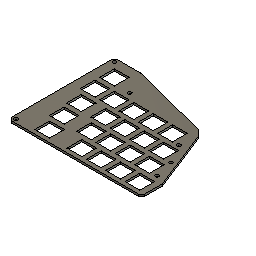
Main Plate v4 (Autodesk Fusion 360 design; units mm, degrees)
Autodesk Fusion 360 part; units mm, degrees
other "Base Mesh Feature1"
sketch "Sketch1" plane through (0, 0, 0) normal (0, 1, 0) x (1, 0, 0)
  line L0 (2.5, 38.25) -> (0, 40.75)
  line L1 (0, 40.75) -> (0, 136)
  line L2 (0, 136) -> (0, 138.5)
  line L3 (0, 138.5) -> (2.5, 138.5)
  line L4 (2.5, 138.5) -> (0, 136)
  line L5 (2.5, 138.5) -> (25, 138.5)
  line L6 (96.5, 117.5) -> (98.5, 117.5)
  line L7 (98.5, 117.5) -> (98.5, 119.5)
  line L8 (98.5, 119.5) -> (25, 138.5)
  line L9 (102, 112) -> (104, 112)
  line L10 (104, 112) -> (104, 114)
  line L11 (104, 114) -> (98.5, 119.5)
  line L12 (2.5, 38.25) -> (121.5, 38.25)
  line L13 (121.5, 38.25) -> (123.5, 38.25)
  line L14 (123.5, 38.25) -> (126, 38.25)
  line L15 (126, 38.25) -> (126, 40.75)
  line L16 (126, 40.75) -> (123.5, 38.25)
  line L17 (124, 58) -> (126, 58)
  line L18 (126, 58) -> (126, 40.75)
  line L19 (126, 58) -> (104, 114)
  dimension "d1" = 95.25
  dimension "d2" = 2.5
  dimension "d3" = 2.5
  dimension "d4" = 2
  dimension "d5" = 2
  dimension "d6" = 2
  dimension "d7" = 2
  dimension "d8" = 2.5
  dimension "d9" = 2.5
  constraint vertical L1
  constraint parallel L1 L2
  constraint perpendicular L2 L3
  constraint perpendicular L1 L5
  constraint perpendicular L1 L6
  constraint perpendicular L6 L7
  constraint perpendicular L7 L9
  constraint perpendicular L9 L10
  constraint horizontal L12
  constraint parallel L12 L13
  constraint parallel L13 L14
  constraint perpendicular L14 L15
  constraint parallel L13 L17
  constraint perpendicular L17 L18
  measures "d1" distance of L0.end L1.end
  measures "d2" distance of L1.end L2.end
  measures "d3" distance of L2.end L3.end
  measures "d4" distance of L6.start L6.end
  measures "d5" distance of L6.end L7.end
  measures "d6" distance of L9.start L9.end
  measures "d7" distance of L12.end L13.end
  measures "d8" distance of L13.end L14.end
  measures "d9" distance of L14.end L15.end
extrude "Extrude1" add sketch "Sketch1" against normal blind 2 contours L0 L1 L4 L5 L8 L11 L12 L13 L16 L18 L19
sketch "Sketch2" plane through (0, 0, 0) normal (0, 1, 0) x (-1, 0, 0)
  line L0 (-126, -40.75) -> (-126, -58)
  line L1 (-126, -58) -> (-104, -114)
  line L2 (-104, -114) -> (-98.5, -119.5)
  line L3 (-98.5, -119.5) -> (-25, -138.5)
  line L4 (-25, -138.5) -> (-2.5, -138.5)
  line L5 (-2.5, -138.5) -> (0, -136)
  line L6 (0, -136) -> (0, -40.75)
  line L7 (0, -40.75) -> (-2.5, -38.25)
  line L8 (-2.5, -38.25) -> (-123.5, -38.25)
  line L9 (-123.5, -38.25) -> (-126, -40.75)
  line L10 (-3.5, -40.125) -> (-3.5, -41.75)
  circle A0 centre (-3.5, -41.75) radius 1.625
  line L11 (0, -138.5) -> (-3.45, -138.5)
  line L12 (-3.45, -138.5) -> (-3.45, -135.05)
  circle A1 centre (-3.45, -135.05) radius 1.625
  dimension "d12" = 1.625
  dimension "d13" = 3.45
  dimension "d14" = 3.45
  dimension "d15" = 3.25
  constraint vertical L10
  constraint coincident L10.end A0.centre
  constraint coincident L10.start A0
  constraint parallel L4 L11
  constraint perpendicular L11 L12
  constraint coincident L12.end A1.centre
  measures "d12" distance of L10.start L10.end
  measures "d13" distance of L11.start L11.end
  measures "d14" distance of L11.end L12.end
  measures "d15" diameter of A1
extrude "Extrude2" cut sketch "Sketch2" against normal blind 2 contours A0 | A1
move_body "Move1" bodies 1 to x (1, 0, 0) y (0, 1, 0) z (0, 0, 1) at (0, 0, 38.25)
sketch "Sketch3" plane through (0, 0, 0) normal (0, 1, 0) x (-1, 0, 0)
  circle A0 centre (-3.45, -96.8) radius 1.625
  circle A1 centre (-3.5, -3.5) radius 1.625
  line L0 (-126, -2.5) -> (-126, -19.75)
  line L1 (-126, -19.75) -> (-104, -75.75)
  line L2 (-104, -75.75) -> (-98.5, -81.25)
  line L3 (-98.5, -81.25) -> (-25, -100.25)
  line L4 (-25, -100.25) -> (-2.5, -100.25)
  line L5 (-2.5, -100.25) -> (0, -97.75)
  line L6 (0, -97.75) -> (0, -2.5)
  line L7 (0, -2.5) -> (-2.5, 0)
  line L8 (-2.5, 0) -> (-123.5, 0)
  line L9 (-123.5, 0) -> (-126, -2.5)
  line L10 (-21.075, -3.85) -> (-35.075, -3.85)
  line L11 (-35.075, -3.85) -> (-35.075, -17.85)
  line L12 (-35.075, -17.85) -> (-21.075, -17.85)
  line L13 (-21.075, -17.85) -> (-21.075, -3.85)
  line L14 (-51, -3.85) -> (-51.5, -3.85)
  line L15 (-51.5, -3.85) -> (-65.5, -3.85)
  line L16 (-65.5, -3.85) -> (-65.5, -17.85)
  line L17 (-65.5, -17.85) -> (-51.5, -17.85)
  line L18 (-51.5, -17.85) -> (-51.5, -3.85)
  line L19 (-65.5, -3.85) -> (-83.85, -3.85)
  line L20 (-83.85, -3.85) -> (-69.85, -3.85)
  line L21 (-69.85, -3.85) -> (-69.85, -17.85)
  line L22 (-69.85, -17.85) -> (-83.85, -17.85)
  line L23 (-83.85, -17.85) -> (-83.85, -3.85)
  line L24 (-83.85, -3.85) -> (-102.2, -3.85)
  line L25 (-102.2, -3.85) -> (-88.2, -3.85)
  line L26 (-88.2, -3.85) -> (-88.2, -17.85)
  line L27 (-88.2, -17.85) -> (-102.2, -17.85)
  line L28 (-102.2, -17.85) -> (-102.2, -3.85)
  line L29 (-102.2, -3.85) -> (-120.55, -3.85)
  line L30 (-120.55, -3.85) -> (-106.55, -3.85)
  line L31 (-106.55, -3.85) -> (-106.55, -17.85)
  line L32 (-106.55, -17.85) -> (-120.55, -17.85)
  line L33 (-120.55, -17.85) -> (-120.55, -3.85)
  dimension "d18" = 14
  dimension "d19" = 14
  dimension "d20" = 0.5
  dimension "d21" = 14
  dimension "d22" = 14
  dimension "d23" = 18.35
  dimension "d24" = 14
  dimension "d25" = 14
  dimension "d26" = 18.35
  dimension "d27" = 14
  dimension "d28" = 14
  dimension "d29" = 18.35
  dimension "d30" = 14
  dimension "d31" = 14
  constraint horizontal L10
  constraint vertical L11
  constraint horizontal L12
  constraint vertical L13
  constraint horizontal L14
  constraint horizontal L15
  constraint vertical L16
  constraint horizontal L17
  constraint vertical L18
  constraint perpendicular L16 L19
  constraint horizontal L20
  constraint vertical L21
  constraint horizontal L22
  constraint vertical L23
  constraint perpendicular L23 L24
  constraint horizontal L25
  constraint vertical L26
  constraint horizontal L27
  constraint vertical L28
  constraint perpendicular L28 L29
  constraint horizontal L30
  constraint vertical L31
  constraint horizontal L32
  constraint vertical L33
  measures "d18" distance of L10.start L10.end
  measures "d19" distance of L10.start L12.end
  measures "d20" distance of L14.start L14.end
  measures "d21" distance of L14.end L15.end
  measures "d22" distance of L14.end L17.end
  measures "d23" distance of L15.end L19.end
  measures "d24" distance of L19.end L20.end
  measures "d25" distance of L19.end L22.end
  measures "d26" distance of L19.end L24.end
  measures "d27" distance of L24.end L25.end
  measures "d28" distance of L24.end L27.end
  measures "d29" distance of L24.end L29.end
  measures "d30" distance of L29.end L30.end
  measures "d31" distance of L29.end L32.end
extrude "Extrude3" cut sketch "Sketch3" against normal blind 2 contours L10 L11 L12 L13 | L15 L16 L17 L18 | L19 L20 L21 L22 L23 | L24 L25 L26 L27 L28 | L29 L30 L31 L32 L33
sketch "Sketch4" plane through (0, 0, 0) normal (0, 1, 0) x (1, 0, 0)
  line L0 (16.5, 21.725) -> (16.5, 22.225)
  line L1 (16.5, 22.225) -> (30.5, 22.225)
  line L2 (30.5, 22.225) -> (30.5, 36.225)
  line L3 (30.5, 36.225) -> (16.5, 36.225)
  line L4 (16.5, 36.225) -> (16.5, 22.225)
  line L5 (41.675, 21.725) -> (42.175, 21.725)
  line L6 (42.175, 21.725) -> (42.175, 22.225)
  line L7 (42.175, 22.225) -> (41.675, 22.225)
  line L8 (41.675, 22.225) -> (41.675, 21.725)
  line L9 (42.175, 22.225) -> (56.175, 22.225)
  line L10 (56.175, 22.225) -> (56.175, 36.225)
  line L11 (56.175, 36.225) -> (42.175, 36.225)
  line L12 (42.175, 36.225) -> (42.175, 22.225)
  line L13 (56.175, 22.225) -> (74.525, 22.225)
  line L14 (74.525, 22.225) -> (60.525, 22.225)
  line L15 (60.525, 22.225) -> (60.525, 36.225)
  line L16 (60.525, 36.225) -> (74.525, 36.225)
  line L17 (74.525, 36.225) -> (74.525, 22.225)
  line L18 (74.525, 22.225) -> (92.875, 22.225)
  line L19 (92.875, 22.225) -> (78.875, 22.225)
  line L20 (78.875, 22.225) -> (78.875, 36.225)
  line L21 (78.875, 36.225) -> (92.875, 36.225)
  line L22 (92.875, 36.225) -> (92.875, 22.225)
  line L23 (92.875, 22.225) -> (111.225, 22.225)
  line L24 (111.225, 22.225) -> (97.225, 22.225)
  line L25 (97.225, 22.225) -> (97.225, 36.225)
  line L26 (97.225, 36.225) -> (111.225, 36.225)
  line L27 (111.225, 36.225) -> (111.225, 22.225)
  line L28 (113.375, 23.75) -> (115.5, 23.75)
  circle A0 centre (115.5, 23.75) radius 1.625
  dimension "d34" = 0.5
  dimension "d35" = 14
  dimension "d36" = 14
  dimension "d37" = 0.5
  dimension "d38" = 0.5
  dimension "d39" = 14
  dimension "d40" = 14
  dimension "d41" = 18.35
  dimension "d42" = 14
  dimension "d43" = 14
  dimension "d44" = 18.35
  dimension "d45" = 14
  dimension "d46" = 14
  dimension "d47" = 18.35
  dimension "d48" = 14
  dimension "d49" = 14
  dimension "d50" = 2.125
  dimension "d51" = 3.25
  constraint vertical L0
  constraint horizontal L1
  constraint vertical L2
  constraint horizontal L3
  constraint vertical L4
  constraint horizontal L5
  constraint vertical L6
  constraint horizontal L7
  constraint vertical L8
  constraint horizontal L9
  constraint vertical L10
  constraint horizontal L11
  constraint vertical L12
  constraint perpendicular L10 L13
  constraint horizontal L14
  constraint vertical L15
  constraint horizontal L16
  constraint vertical L17
  constraint perpendicular L17 L18
  constraint horizontal L19
  constraint vertical L20
  constraint horizontal L21
  constraint vertical L22
  constraint perpendicular L22 L23
  constraint horizontal L24
  constraint vertical L25
  constraint horizontal L26
  constraint vertical L27
  constraint horizontal L28
  constraint coincident L28.end A0.centre
  measures "d34" distance of L0.start L0.end
  measures "d35" distance of L0.end L1.end
  measures "d36" distance of L0.end L3.end
  measures "d37" distance of L5.start L5.end
  measures "d38" distance of L5.start L7.end
  measures "d39" distance of L6.end L9.end
  measures "d40" distance of L6.end L11.end
  measures "d41" distance of L9.end L13.end
  measures "d42" distance of L13.end L14.end
  measures "d43" distance of L13.end L16.end
  measures "d44" distance of L13.end L18.end
  measures "d45" distance of L18.end L19.end
  measures "d46" distance of L18.end L21.end
  measures "d47" distance of L18.end L23.end
  measures "d48" distance of L23.end L24.end
  measures "d49" distance of L23.end L26.end
  measures "d50" distance of L28.start L28.end
  measures "d51" diameter of A0
extrude "Extrude4" cut sketch "Sketch4" against normal blind 2 contours L1 L2 L3 L4 | L9 L10 L11 L12 | L13 L14 L15 L16 L17 | L18 L19 L20 L21 L22 | L23 L24 L25 L26 L27 | A0
sketch "Sketch5" plane through (0, 0, 0) normal (0, 1, 0) x (-1, 0, 0)
  line L0 (-78.875, -22.225) -> (-78.875, -36.225)
  line L1 (-78.875, -36.225) -> (-92.875, -36.225)
  line L2 (-92.875, -36.225) -> (-92.875, -22.225)
  line L3 (-92.875, -22.225) -> (-78.875, -22.225)
  line L4 (-30.5, -22.225) -> (-16.5, -22.225)
  line L5 (-16.5, -22.225) -> (-16.5, -36.225)
  line L6 (-16.5, -36.225) -> (-30.5, -36.225)
  line L7 (-30.5, -36.225) -> (-30.5, -22.225)
  line L8 (-97.225, -22.225) -> (-97.225, -36.225)
  line L9 (-97.225, -36.225) -> (-111.225, -36.225)
  line L10 (-111.225, -36.225) -> (-111.225, -22.225)
  line L11 (-111.225, -22.225) -> (-97.225, -22.225)
  line L12 (-60.525, -22.225) -> (-60.525, -36.225)
  line L13 (-60.525, -36.225) -> (-74.525, -36.225)
  line L14 (-74.525, -36.225) -> (-74.525, -22.225)
  line L15 (-74.525, -22.225) -> (-60.525, -22.225)
  line L16 (-56.175, -22.225) -> (-42.175, -22.225)
  line L17 (-42.175, -22.225) -> (-42.175, -36.225)
  line L18 (-42.175, -36.225) -> (-56.175, -36.225)
  line L19 (-56.175, -36.225) -> (-56.175, -22.225)
  circle A0 centre (-115.5, -23.75) radius 1.625
  line L20 (-69.85, -3.85) -> (-69.85, -17.85)
  line L21 (-69.85, -17.85) -> (-83.85, -17.85)
  line L22 (-83.85, -17.85) -> (-83.85, -3.85)
  line L23 (-83.85, -3.85) -> (-69.85, -3.85)
  line L24 (-88.2, -3.85) -> (-88.2, -17.85)
  line L25 (-88.2, -17.85) -> (-102.2, -17.85)
  line L26 (-102.2, -17.85) -> (-102.2, -3.85)
  line L27 (-102.2, -3.85) -> (-88.2, -3.85)
  line L28 (-65.5, -3.85) -> (-51.5, -3.85)
  line L29 (-51.5, -3.85) -> (-51.5, -17.85)
  line L30 (-51.5, -17.85) -> (-65.5, -17.85)
  line L31 (-65.5, -17.85) -> (-65.5, -3.85)
  line L32 (-106.55, -3.85) -> (-106.55, -17.85)
  line L33 (-106.55, -17.85) -> (-120.55, -17.85)
  line L34 (-120.55, -17.85) -> (-120.55, -3.85)
  line L35 (-120.55, -3.85) -> (-106.55, -3.85)
  line L36 (-35.075, -3.85) -> (-21.075, -3.85)
  line L37 (-21.075, -3.85) -> (-21.075, -17.85)
  line L38 (-21.075, -17.85) -> (-35.075, -17.85)
  line L39 (-35.075, -17.85) -> (-35.075, -3.85)
  circle A1 centre (-3.45, -96.8) radius 1.625
  circle A2 centre (-3.5, -3.5) radius 1.625
  line L40 (-126, -2.5) -> (-126, -19.75)
  line L41 (-126, -19.75) -> (-104, -75.75)
  line L42 (-104, -75.75) -> (-98.5, -81.25)
  line L43 (-98.5, -81.25) -> (-25, -100.25)
  line L44 (-25, -100.25) -> (-2.5, -100.25)
  line L45 (-2.5, -100.25) -> (0, -97.75)
  line L46 (0, -97.75) -> (0, -2.5)
  line L47 (0, -2.5) -> (-2.5, 0)
  line L48 (-2.5, 0) -> (-123.5, 0)
  line L49 (-123.5, 0) -> (-126, -2.5)
  line L50 (-14.325, -39.6) -> (-14.325, -40.6)
  line L51 (-14.325, -40.6) -> (-28.325, -40.6)
  line L52 (-28.325, -40.6) -> (-28.325, -54.6)
  line L53 (-28.325, -54.6) -> (-14.325, -54.6)
  line L54 (-14.325, -54.6) -> (-14.325, -40.6)
  line L55 (-36.75, -39.6) -> (-37.25, -39.6)
  line L56 (-37.25, -39.6) -> (-37.25, -40.6)
  line L57 (-37.25, -40.6) -> (-36.75, -40.6)
  line L58 (-36.75, -40.6) -> (-36.75, -39.6)
  line L59 (-37.25, -40.6) -> (-51.25, -40.6)
  line L60 (-51.25, -40.6) -> (-51.25, -54.6)
  line L61 (-51.25, -54.6) -> (-37.25, -54.6)
  line L62 (-37.25, -54.6) -> (-37.25, -40.6)
  line L63 (-51.25, -40.6) -> (-69.6, -40.6)
  line L64 (-69.6, -40.6) -> (-55.6, -40.6)
  line L65 (-55.6, -40.6) -> (-55.6, -54.6)
  line L66 (-55.6, -54.6) -> (-69.6, -54.6)
  line L67 (-69.6, -54.6) -> (-69.6, -40.6)
  line L68 (-69.6, -40.6) -> (-87.95, -40.6)
  line L69 (-87.95, -40.6) -> (-73.95, -40.6)
  line L70 (-73.95, -40.6) -> (-73.95, -54.6)
  line L71 (-73.95, -54.6) -> (-87.95, -54.6)
  line L72 (-87.95, -54.6) -> (-87.95, -40.6)
  line L73 (-87.95, -40.6) -> (-106.3, -40.6)
  line L74 (-106.3, -40.6) -> (-92.3, -40.6)
  line L75 (-92.3, -40.6) -> (-92.3, -54.6)
  line L76 (-92.3, -54.6) -> (-106.3, -54.6)
  line L77 (-106.3, -54.6) -> (-106.3, -40.6)
  line L78 (-108.875, -41.25) -> (-111, -41.25)
  line L79 (-111, -41.25) -> (-112.5, -41.25)
  circle A3 centre (-112.5, -41.25) radius 1.625
  line L80 (-115.5, -23.75) -> (-117, -23.75)
  circle A4 centre (-117, -23.75) radius 1.625
  dimension "d54" = 1
  dimension "d55" = 14
  dimension "d56" = 14
  dimension "d57" = 0.5
  dimension "d58" = 1
  dimension "d59" = 14
  dimension "d60" = 14
  dimension "d61" = 18.35
  dimension "d62" = 14
  dimension "d63" = 14
  dimension "d64" = 18.35
  dimension "d65" = 14
  dimension "d66" = 14
  dimension "d67" = 18.35
  dimension "d68" = 14
  dimension "d69" = 14
  dimension "d70" = 2.125
  dimension "d71" = 1.5
  dimension "d72" = 3.25
  dimension "d73" = 1.5
  dimension "d74" = 3.25
  constraint vertical L50
  constraint horizontal L51
  constraint vertical L52
  constraint horizontal L53
  constraint vertical L54
  constraint horizontal L55
  constraint vertical L56
  constraint horizontal L57
  constraint vertical L58
  constraint horizontal L59
  constraint vertical L60
  constraint horizontal L61
  constraint vertical L62
  constraint perpendicular L60 L63
  constraint horizontal L64
  constraint vertical L65
  constraint horizontal L66
  constraint vertical L67
  constraint perpendicular L67 L68
  constraint horizontal L69
  constraint vertical L70
  constraint horizontal L71
  constraint vertical L72
  constraint perpendicular L72 L73
  constraint horizontal L74
  constraint vertical L75
  constraint horizontal L76
  constraint vertical L77
  constraint horizontal L78
  constraint parallel L78 L79
  constraint coincident L79.end A3.centre
  constraint coincident A0.centre L80.start
  constraint horizontal L80
  constraint coincident L80.end A4.centre
  measures "d54" distance of L50.start L50.end
  measures "d55" distance of L50.end L51.end
  measures "d56" distance of L50.end L53.end
  measures "d57" distance of L55.start L55.end
  measures "d58" distance of L55.start L57.end
  measures "d59" distance of L56.end L59.end
  measures "d60" distance of L56.end L61.end
  measures "d61" distance of L59.end L63.end
  measures "d62" distance of L63.end L64.end
  measures "d63" distance of L63.end L66.end
  measures "d64" distance of L63.end L68.end
  measures "d65" distance of L68.end L69.end
  measures "d66" distance of L68.end L71.end
  measures "d67" distance of L68.end L73.end
  measures "d68" distance of L73.end L74.end
  measures "d69" distance of L73.end L76.end
  measures "d70" distance of L78.start L78.end
  measures "d71" distance of L78.end L79.end
  measures "d72" diameter of A3
  measures "d73" distance of A0.centre L80.end
  measures "d74" diameter of A4
extrude "Extrude5" cut sketch "Sketch5" against normal blind 2 contours A0 A4 | A0 A4 | L51 L52 L53 L54 | L59 L60 L61 L62 | L63 L64 L65 L66 L67 | L68 L69 L70 L71 L72 | L73 L74 L75 L76 L77 | A3 picked at (-116.5388, -23.75) picked at (-118.049, -23.3238)
sketch "Sketch6" plane through (0, 0, 0) normal (0, 1, 0) x (-1, 0, 0)
  line L0 (-126, -2.5) -> (-126, -19.75)
  line L1 (-126, -19.75) -> (-104, -75.75)
  line L2 (-104, -75.75) -> (-98.5, -81.25)
  line L3 (-98.5, -81.25) -> (-25, -100.25)
  line L4 (-25, -100.25) -> (-2.5, -100.25)
  line L5 (-2.5, -100.25) -> (0, -97.75)
  line L6 (0, -97.75) -> (0, -2.5)
  line L7 (0, -2.5) -> (-2.5, 0)
  line L8 (-2.5, 0) -> (-123.5, 0)
  line L9 (-123.5, 0) -> (-126, -2.5)
  circle A0 centre (-3.5, -3.5) radius 1.625
  circle A1 centre (-3.45, -96.8) radius 1.625
  line L10 (-35.075, -3.85) -> (-21.075, -3.85)
  line L11 (-21.075, -3.85) -> (-21.075, -17.85)
  line L12 (-21.075, -17.85) -> (-35.075, -17.85)
  line L13 (-35.075, -17.85) -> (-35.075, -3.85)
  line L14 (-106.55, -3.85) -> (-106.55, -17.85)
  line L15 (-106.55, -17.85) -> (-120.55, -17.85)
  line L16 (-120.55, -17.85) -> (-120.55, -3.85)
  line L17 (-120.55, -3.85) -> (-106.55, -3.85)
  line L18 (-65.5, -3.85) -> (-51.5, -3.85)
  line L19 (-51.5, -3.85) -> (-51.5, -17.85)
  line L20 (-51.5, -17.85) -> (-65.5, -17.85)
  line L21 (-65.5, -17.85) -> (-65.5, -3.85)
  line L22 (-88.2, -3.85) -> (-88.2, -17.85)
  line L23 (-88.2, -17.85) -> (-102.2, -17.85)
  line L24 (-102.2, -17.85) -> (-102.2, -3.85)
  line L25 (-102.2, -3.85) -> (-88.2, -3.85)
  line L26 (-69.85, -3.85) -> (-69.85, -17.85)
  line L27 (-69.85, -17.85) -> (-83.85, -17.85)
  line L28 (-83.85, -17.85) -> (-83.85, -3.85)
  line L29 (-83.85, -3.85) -> (-69.85, -3.85)
  arc A2 (-116.25, -22.3084) -> (-116.25, -25.1916) centre (-117, -23.75) ccw
  arc A3 (-116.25, -25.1916) -> (-116.25, -22.3084) centre (-115.5, -23.75) ccw
  line L30 (-56.175, -22.225) -> (-42.175, -22.225)
  line L31 (-42.175, -22.225) -> (-42.175, -36.225)
  line L32 (-42.175, -36.225) -> (-56.175, -36.225)
  line L33 (-56.175, -36.225) -> (-56.175, -22.225)
  line L34 (-60.525, -22.225) -> (-60.525, -36.225)
  line L35 (-60.525, -36.225) -> (-74.525, -36.225)
  line L36 (-74.525, -36.225) -> (-74.525, -22.225)
  line L37 (-74.525, -22.225) -> (-60.525, -22.225)
  line L38 (-97.225, -22.225) -> (-97.225, -36.225)
  line L39 (-97.225, -36.225) -> (-111.225, -36.225)
  line L40 (-111.225, -36.225) -> (-111.225, -22.225)
  line L41 (-111.225, -22.225) -> (-97.225, -22.225)
  line L42 (-30.5, -22.225) -> (-16.5, -22.225)
  line L43 (-16.5, -22.225) -> (-16.5, -36.225)
  line L44 (-16.5, -36.225) -> (-30.5, -36.225)
  line L45 (-30.5, -36.225) -> (-30.5, -22.225)
  line L46 (-78.875, -22.225) -> (-78.875, -36.225)
  line L47 (-78.875, -36.225) -> (-92.875, -36.225)
  line L48 (-92.875, -36.225) -> (-92.875, -22.225)
  line L49 (-92.875, -22.225) -> (-78.875, -22.225)
  line L50 (-28.325, -40.6) -> (-14.325, -40.6)
  line L51 (-14.325, -40.6) -> (-14.325, -54.6)
  line L52 (-14.325, -54.6) -> (-28.325, -54.6)
  line L53 (-28.325, -54.6) -> (-28.325, -40.6)
  line L54 (-92.3, -40.6) -> (-92.3, -54.6)
  line L55 (-92.3, -54.6) -> (-106.3, -54.6)
  line L56 (-106.3, -54.6) -> (-106.3, -40.6)
  line L57 (-106.3, -40.6) -> (-92.3, -40.6)
  circle A4 centre (-112.5, -41.25) radius 1.625
  line L58 (-51.25, -40.6) -> (-37.25, -40.6)
  line L59 (-37.25, -40.6) -> (-37.25, -54.6)
  line L60 (-37.25, -54.6) -> (-51.25, -54.6)
  line L61 (-51.25, -54.6) -> (-51.25, -40.6)
  line L62 (-73.95, -40.6) -> (-73.95, -54.6)
  line L63 (-73.95, -54.6) -> (-87.95, -54.6)
  line L64 (-87.95, -54.6) -> (-87.95, -40.6)
  line L65 (-87.95, -40.6) -> (-73.95, -40.6)
  line L66 (-55.6, -40.6) -> (-55.6, -54.6)
  line L67 (-55.6, -54.6) -> (-69.6, -54.6)
  line L68 (-69.6, -54.6) -> (-69.6, -40.6)
  line L69 (-69.6, -40.6) -> (-55.6, -40.6)
  line L70 (-9, -57.4) -> (-9, -58.9)
  line L71 (-9, -58.9) -> (-23, -58.9)
  line L72 (-23, -58.9) -> (-23, -72.9)
  line L73 (-23, -72.9) -> (-9, -72.9)
  line L74 (-9, -72.9) -> (-9, -58.9)
  line L75 (-23, -58.9) -> (-41.35, -58.9)
  line L76 (-41.35, -58.9) -> (-27.35, -58.9)
  line L77 (-27.35, -58.9) -> (-27.35, -72.9)
  line L78 (-27.35, -72.9) -> (-41.35, -72.9)
  line L79 (-41.35, -72.9) -> (-41.35, -58.9)
  line L80 (-41.35, -58.9) -> (-59.7, -58.9)
  line L81 (-59.7, -58.9) -> (-45.7, -58.9)
  line L82 (-45.7, -58.9) -> (-45.7, -72.9)
  line L83 (-45.7, -72.9) -> (-59.7, -72.9)
  line L84 (-59.7, -72.9) -> (-59.7, -58.9)
  line L85 (-59.7, -58.9) -> (-78.05, -58.9)
  line L86 (-78.05, -58.9) -> (-64.05, -58.9)
  line L87 (-64.05, -58.9) -> (-64.05, -72.9)
  line L88 (-64.05, -72.9) -> (-78.05, -72.9)
  line L89 (-78.05, -72.9) -> (-78.05, -58.9)
  line L90 (-78.05, -58.9) -> (-96.4, -58.9)
  line L91 (-96.4, -58.9) -> (-82.4, -58.9)
  line L92 (-82.4, -58.9) -> (-82.4, -72.9)
  line L93 (-82.4, -72.9) -> (-96.4, -72.9)
  line L94 (-96.4, -72.9) -> (-96.4, -58.9)
  line L95 (-98.375, -59.25) -> (-102, -59.25)
  circle A5 centre (-102, -59.25) radius 1.625
  line L96 (-9, -75.25) -> (-9, -77.25)
  line L97 (-9, -77.25) -> (-23, -77.25)
  line L98 (-23, -77.25) -> (-23, -91.25)
  line L99 (-23, -91.25) -> (-9, -91.25)
  line L100 (-9, -91.25) -> (-9, -77.25)
  line L101 (0, 0) -> (-36, 0)
  line L102 (-36, 0) -> (-36, -78.75)
  circle A6 centre (-36, -78.75) radius 1.625
  dimension "d77" = 1.5
  dimension "d78" = 14
  dimension "d79" = 14
  dimension "d80" = 18.35
  dimension "d81" = 14
  dimension "d82" = 14
  dimension "d83" = 18.35
  dimension "d84" = 14
  dimension "d85" = 14
  dimension "d86" = 18.35
  dimension "d87" = 14
  dimension "d88" = 14
  dimension "d89" = 18.35
  dimension "d90" = 14
  dimension "d91" = 14
  dimension "d92" = 3.625
  dimension "d93" = 3.25
  dimension "d94" = 2
  dimension "d95" = 14
  dimension "d96" = 14
  dimension "d97" = 36
  dimension "d98" = 78.75
  dimension "d99" = 3.25
  constraint perpendicular L52 L70
  constraint horizontal L71
  constraint vertical L72
  constraint horizontal L73
  constraint vertical L74
  constraint perpendicular L72 L75
  constraint horizontal L76
  constraint vertical L77
  constraint horizontal L78
  constraint vertical L79
  constraint perpendicular L79 L80
  constraint horizontal L81
  constraint vertical L82
  constraint horizontal L83
  constraint vertical L84
  constraint perpendicular L84 L85
  constraint horizontal L86
  constraint vertical L87
  constraint horizontal L88
  constraint vertical L89
  constraint perpendicular L89 L90
  constraint horizontal L91
  constraint vertical L92
  constraint horizontal L93
  constraint vertical L94
  constraint horizontal L95
  constraint coincident L95.end A5.centre
  constraint vertical L96
  constraint horizontal L97
  constraint vertical L98
  constraint horizontal L99
  constraint vertical L100
  constraint coincident L101.start origin
  constraint parallel L8 L101
  constraint vertical L102
  constraint coincident L102.end A6.centre
  measures "d77" distance of L70.start L70.end
  measures "d78" distance of L70.end L71.end
  measures "d79" distance of L70.end L73.end
  measures "d80" distance of L71.end L75.end
  measures "d81" distance of L75.end L76.end
  measures "d82" distance of L75.end L78.end
  measures "d83" distance of L75.end L80.end
  measures "d84" distance of L80.end L81.end
  measures "d85" distance of L80.end L83.end
  measures "d86" distance of L80.end L85.end
  measures "d87" distance of L85.end L86.end
  measures "d88" distance of L85.end L88.end
  measures "d89" distance of L85.end L90.end
  measures "d90" distance of L90.end L91.end
  measures "d91" distance of L90.end L93.end
  measures "d92" distance of L95.start L95.end
  measures "d93" diameter of A5
  measures "d94" distance of L96.start L96.end
  measures "d95" distance of L96.end L97.end
  measures "d96" distance of L96.end L99.end
  measures "d97" distance of L101.start L101.end
  measures "d98" distance of L101.end L102.end
  measures "d99" diameter of A6
extrude "Extrude6" cut sketch "Sketch6" against normal blind 2 contours L71 L72 L73 L74 | L75 L76 L77 L78 L102 | L75 L76 L78 L79 L102 | L80 L81 L82 L83 L84 | L85 L86 L87 L88 L89 | L90 L91 L92 L93 L94 | A5 | L97 L98 L99 L100 | A6
sketch "Sketch7" plane through (0, 0, 0) normal (0, 1, 0) x (-1, 0, 0)
  line L0 (-64.05, -58.9) -> (-64.05, -72.9)
  line L1 (-64.05, -72.9) -> (-78.05, -72.9)
  line L2 (-78.05, -72.9) -> (-78.05, -58.9)
  line L3 (-78.05, -58.9) -> (-64.05, -58.9)
  line L4 (-23, -77.25) -> (-9, -77.25)
  line L5 (-9, -77.25) -> (-9, -91.25)
  line L6 (-9, -91.25) -> (-23, -91.25)
  line L7 (-23, -91.25) -> (-23, -77.25)
  circle A0 centre (-36, -78.75) radius 1.625
  line L8 (-82.4, -58.9) -> (-82.4, -72.9)
  line L9 (-82.4, -72.9) -> (-96.4, -72.9)
  line L10 (-96.4, -72.9) -> (-96.4, -58.9)
  line L11 (-96.4, -58.9) -> (-82.4, -58.9)
  line L12 (-45.7, -58.9) -> (-45.7, -72.9)
  line L13 (-45.7, -72.9) -> (-59.7, -72.9)
  line L14 (-59.7, -72.9) -> (-59.7, -58.9)
  line L15 (-59.7, -58.9) -> (-45.7, -58.9)
  line L16 (-23, -58.9) -> (-9, -58.9)
  line L17 (-9, -58.9) -> (-9, -72.9)
  line L18 (-9, -72.9) -> (-23, -72.9)
  line L19 (-23, -72.9) -> (-23, -58.9)
  line L20 (-27.35, -58.9) -> (-27.35, -72.9)
  line L21 (-27.35, -72.9) -> (-41.35, -72.9)
  line L22 (-41.35, -72.9) -> (-41.35, -58.9)
  line L23 (-41.35, -58.9) -> (-27.35, -58.9)
  circle A1 centre (-102, -59.25) radius 1.625
  line L24 (-126, -2.5) -> (-126, -19.75)
  line L25 (-126, -19.75) -> (-104, -75.75)
  line L26 (-104, -75.75) -> (-98.5, -81.25)
  line L27 (-98.5, -81.25) -> (-25, -100.25)
  line L28 (-25, -100.25) -> (-2.5, -100.25)
  line L29 (-2.5, -100.25) -> (0, -97.75)
  line L30 (0, -97.75) -> (0, -2.5)
  line L31 (0, -2.5) -> (-2.5, 0)
  line L32 (-2.5, 0) -> (-123.5, 0)
  line L33 (-123.5, 0) -> (-126, -2.5)
  circle A2 centre (-3.5, -3.5) radius 1.625
  circle A3 centre (-3.45, -96.8) radius 1.625
  line L34 (-35.075, -3.85) -> (-21.075, -3.85)
  line L35 (-21.075, -3.85) -> (-21.075, -17.85)
  line L36 (-21.075, -17.85) -> (-35.075, -17.85)
  line L37 (-35.075, -17.85) -> (-35.075, -3.85)
  line L38 (-106.55, -3.85) -> (-106.55, -17.85)
  line L39 (-106.55, -17.85) -> (-120.55, -17.85)
  line L40 (-120.55, -17.85) -> (-120.55, -3.85)
  line L41 (-120.55, -3.85) -> (-106.55, -3.85)
  line L42 (-65.5, -3.85) -> (-51.5, -3.85)
  line L43 (-51.5, -3.85) -> (-51.5, -17.85)
  line L44 (-51.5, -17.85) -> (-65.5, -17.85)
  line L45 (-65.5, -17.85) -> (-65.5, -3.85)
  line L46 (-88.2, -3.85) -> (-88.2, -17.85)
  line L47 (-88.2, -17.85) -> (-102.2, -17.85)
  line L48 (-102.2, -17.85) -> (-102.2, -3.85)
  line L49 (-102.2, -3.85) -> (-88.2, -3.85)
  line L50 (-69.85, -3.85) -> (-69.85, -17.85)
  line L51 (-69.85, -17.85) -> (-83.85, -17.85)
  line L52 (-83.85, -17.85) -> (-83.85, -3.85)
  line L53 (-83.85, -3.85) -> (-69.85, -3.85)
  arc A4 (-116.25, -22.3084) -> (-116.25, -25.1916) centre (-117, -23.75) ccw
  arc A5 (-116.25, -25.1916) -> (-116.25, -22.3084) centre (-115.5, -23.75) ccw
  line L54 (-56.175, -22.225) -> (-42.175, -22.225)
  line L55 (-42.175, -22.225) -> (-42.175, -36.225)
  line L56 (-42.175, -36.225) -> (-56.175, -36.225)
  line L57 (-56.175, -36.225) -> (-56.175, -22.225)
  line L58 (-60.525, -22.225) -> (-60.525, -36.225)
  line L59 (-60.525, -36.225) -> (-74.525, -36.225)
  line L60 (-74.525, -36.225) -> (-74.525, -22.225)
  line L61 (-74.525, -22.225) -> (-60.525, -22.225)
  line L62 (-97.225, -22.225) -> (-97.225, -36.225)
  line L63 (-97.225, -36.225) -> (-111.225, -36.225)
  line L64 (-111.225, -36.225) -> (-111.225, -22.225)
  line L65 (-111.225, -22.225) -> (-97.225, -22.225)
  line L66 (-30.5, -22.225) -> (-16.5, -22.225)
  line L67 (-16.5, -22.225) -> (-16.5, -36.225)
  line L68 (-16.5, -36.225) -> (-30.5, -36.225)
  line L69 (-30.5, -36.225) -> (-30.5, -22.225)
  line L70 (-78.875, -22.225) -> (-78.875, -36.225)
  line L71 (-78.875, -36.225) -> (-92.875, -36.225)
  line L72 (-92.875, -36.225) -> (-92.875, -22.225)
  line L73 (-92.875, -22.225) -> (-78.875, -22.225)
  line L74 (-28.325, -40.6) -> (-14.325, -40.6)
  line L75 (-14.325, -40.6) -> (-14.325, -54.6)
  line L76 (-14.325, -54.6) -> (-28.325, -54.6)
  line L77 (-28.325, -54.6) -> (-28.325, -40.6)
  line L78 (-92.3, -40.6) -> (-92.3, -54.6)
  line L79 (-92.3, -54.6) -> (-106.3, -54.6)
  line L80 (-106.3, -54.6) -> (-106.3, -40.6)
  line L81 (-106.3, -40.6) -> (-92.3, -40.6)
  circle A6 centre (-112.5, -41.25) radius 1.625
  line L82 (-51.25, -40.6) -> (-37.25, -40.6)
  line L83 (-37.25, -40.6) -> (-37.25, -54.6)
  line L84 (-37.25, -54.6) -> (-51.25, -54.6)
  line L85 (-51.25, -54.6) -> (-51.25, -40.6)
  line L86 (-73.95, -40.6) -> (-73.95, -54.6)
  line L87 (-73.95, -54.6) -> (-87.95, -54.6)
  line L88 (-87.95, -54.6) -> (-87.95, -40.6)
  line L89 (-87.95, -40.6) -> (-73.95, -40.6)
  line L90 (-55.6, -40.6) -> (-55.6, -54.6)
  line L91 (-55.6, -54.6) -> (-69.6, -54.6)
  line L92 (-69.6, -54.6) -> (-69.6, -40.6)
  line L93 (-69.6, -40.6) -> (-55.6, -40.6)
  circle A7 centre (-117, -23.75) radius 1.625
  constraint concentric A4 A7
  constraint coincident A4.end A7
extrude "Extrude7" add sketch "Sketch7" against normal blind 2 contours A5 A7
extrude "Extrude8" cut 1 faces at (62.5167, 0, -84.8) along direction (0, -1, 0) blind 0.1
equation "d12 = ( 3.25 / 2 ) * 1 mm"
equation "d23 = 17.85 mm + 0.5 mm"
equation "d26 = 17.85 mm + 0.5 mm"
equation "d50 = ( 3.25 / 2 ) * 1 mm + 0.5 mm"
equation "d70 = ( 3.25 / 2 ) * 1 mm + 0.5 mm"
equation "d92 = ( 3.25 / 2 ) * 1 mm + 2 mm"
